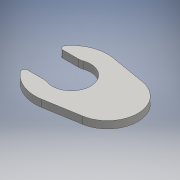
# Autodesk Inventor part: BowdenConnectorPlayClip
Saved by Autodesk Inventor 2016 (Build 200138000, 138)
## iProperties
Created: 2015-05-25
Part Number: BowdenConnectorPlayClip
Material: Generic
Document SubType Name: Modeling
Designer: Jack
Density: 1 g/cm^3
Appearance: Default
Author: Jack
Autodesk Inventor part; units mm, degrees
ref_plane "YZ Plane" through (0, 0, 0) normal (1, 0, 0) x (0, 1, 0)
ref_plane "XZ Plane" through (0, 0, 0) normal (0, 1, 0) x (-1, 0, 0)
ref_plane "XY Plane" through (0, 0, 0) normal (0, 0, 1) x (1, 0, 0)
sketch "Sketch1" plane through (0, 0, 0) normal (0, 0, 1) x (1, 0, 0)
  arc A0 (-1.3528, -2.9) -> (-1.3528, 2.9) centre (0, 0) ccw
  arc A1 (-5.2526, -2.9) -> (-5.2526, 2.9) centre (0, 0) ccw
  line L0 (-1.3528, 2.9) -> (-5.2526, 2.9)
  line L1 (-1.3528, -2.9) -> (-5.2526, -2.9)
  dimension "d0" = 6.4
  dimension "d1" = 12
  dimension "d2" = 5.8
  dimension "d3" = 2.9
  constraints: 4 end point, 4 point on circle, 2 centre point, 2 coincident, 2 horizontal
  measures "d0" diameter of A0
  measures "d1" diameter of A1
  measures "d2" distance between parallel lines of L0 L1
  measures "d3" distance from line of point (0, 0) L0
extrude "Extrusion1" add sketch "Sketch1" along normal blind 1.2
fillet "Fillet1" radius 0.5 2 edges at (-5.2526, 2.9, 0.6) (-5.2526, -2.9, 0.6)
fillet "Fillet2" radius 2 2 edges at (-1.3528, 2.9, 0.6) (-1.3528, -2.9, 0.6)
sketch "Sketch2" plane through (0, 0, 1.2) normal (0, 0, 1) x (1, 0, 0)
  arc A0 (-4.7162, -3.7091) -> (-4.7162, 3.7091) centre (0, 0) ccw projected
  arc A1 (6.8333, -4.9301) -> (6.8333, 4.9301) centre (6, 0) ccw
  line L0 (6.8333, 4.9301) -> (1, 5.9161)
  line L1 (6.8333, -4.9301) -> (1, -5.9161)
  dimension "d8" = 10
  constraints: 5 point on circle, 4 end point, 4 tangent, 1 centre point, 1 horizontal alignment
  measures "d8" diameter of A1
extrude "Extrusion2" add sketch "Sketch2" against normal up to surface (1.2 mm away)
equation "\"d3\" = 0.5 * d2"
body "Solid1"
